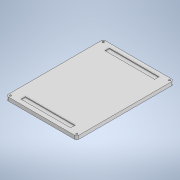
# Autodesk Inventor part: Base Bracket 1x
Saved by Autodesk Inventor 2020.2 (Build 242310000, 310)
## iProperties
Created: 2020-03-30
Part Number: Base Bracket 1x
Material: Generic
Document SubType Name: Modeling
Designer: Amaan Khalid
Density: 1 g/cm^3
Appearance: Default
Author: Amaan Khalid
Autodesk Inventor part; units mm, degrees
ref_plane "YZ Plane" through (0, 0, 0) normal (1, 0, 0) x (0, 1, 0)
ref_plane "XZ Plane" through (0, 0, 0) normal (0, 1, 0) x (-1, 0, 0)
ref_plane "XY Plane" through (0, 0, 0) normal (0, 0, 1) x (1, 0, 0)
sketch "Sketch1" plane through (0, 0, 0) normal (0, 1, 0) x (-1, 0, 0)
  line L0 (163.7334, -183.5335) -> (68.4834, -183.5335)
  line L1 (166.9084, -186.7085) -> (166.9084, -253.3835)
  line L2 (65.3084, -186.7085) -> (65.3084, -253.3835)
  arc A0 (166.9084, -186.7085) -> (163.7334, -183.5335) centre (163.7334, -186.7085) ccw
  arc A1 (68.4834, -183.5335) -> (65.3084, -186.7085) centre (68.4834, -186.7085) ccw
  line L3 (163.7334, -323.2335) -> (68.4834, -323.2335)
  line L4 (166.9084, -320.0585) -> (166.9084, -253.3835)
  line L5 (65.3084, -320.0585) -> (65.3084, -253.3835)
  arc A2 (163.7334, -323.2335) -> (166.9084, -320.0585) centre (163.7334, -320.0585) ccw
  arc A3 (65.3084, -320.0585) -> (68.4834, -323.2335) centre (68.4834, -320.0585) ccw
  point P0 (0, 0)
  point P1 (65.3084, -183.5335)
  dimension "d5" = 69.85
  dimension "d6" = 3.175
  constraints: 12 end point, 8 point on circle, 4 centre point, 4 tangent, 2 point on line, 2 vertical, 1 horizontal
  measures "d5" distance of point (65.308, -183.534) L2.end
  measures "d6" radius of A0
extrude "Extrusion1" add sketch "Sketch1" along normal blind 5.08
sketch "Sketch2" plane through (0, 5.08, 0) normal (0, 1, 0) x (1, 0, 0)
  arc A0 (-166.9084, 186.7085) -> (-163.7334, 183.5335) centre (-163.7334, 186.7085) ccw projected
  circle A1 centre (-163.7334, 186.7085) radius 1.27
  arc A2 (-68.4834, 183.5335) -> (-65.3084, 186.7085) centre (-68.4834, 186.7085) ccw projected
  circle A3 centre (-68.4834, 186.7085) radius 1.27
  arc A4 (-163.7334, 323.2335) -> (-166.9084, 320.0585) centre (-163.7334, 320.0585) ccw projected
  circle A5 centre (-163.7334, 320.0585) radius 1.27
  arc A6 (-65.3084, 320.0585) -> (-68.4834, 323.2335) centre (-68.4834, 320.0585) ccw projected
  circle A7 centre (-68.4834, 320.0585) radius 1.27
  point P0 (0, 0)
  dimension "d11" = 2.54
  dimension "d12" = 2.54
  dimension "d13" = 2.54
  dimension "d14" = 2.54
  constraints: 4 centre point, 4 coincident
  measures "d11" diameter of A1
  measures "d12" diameter of A3
  measures "d13" diameter of A5
  measures "d14" diameter of A7
extrude "Extrusion2" cut sketch "Sketch2" against normal mid plane 25.4
sketch "Sketch3" plane through (0, 5.08, 0) normal (0, 1, 0) x (1, 0, 0)
  line L0 (-68.4834, 323.2335) -> (-163.7334, 323.2335) projected
  line L1 (-116.1084, 316.8835) -> (-80.3833, 316.8835)
  line L2 (-116.1084, 316.8835) -> (-151.8335, 316.8835)
  line L3 (-80.3833, 316.8835) -> (-80.3833, 310.5335)
  line L4 (-80.3833, 310.5335) -> (-151.8335, 310.5335)
  line L5 (-151.8335, 310.5335) -> (-151.8335, 316.8835)
  line L6 (-65.3084, 186.7085) -> (-65.3084, 320.0585) projected
  line L7 (-116.1084, 189.8835) -> (-80.3833, 189.8835)
  line L8 (-116.1084, 189.8835) -> (-151.8335, 189.8835)
  line L9 (-80.3833, 189.8835) -> (-80.3833, 196.2335)
  line L10 (-80.3833, 196.2335) -> (-151.8335, 196.2335)
  line L11 (-151.8335, 196.2335) -> (-151.8335, 189.8835)
  point P0 (0, 0)
  constraints: 20 end point, 2 horizontal, 1 parallel, 1 perpendicular, 1 vertical
extrude "Extrusion3" cut sketch "Sketch3" against normal blind 1.016
body "Solid1"
